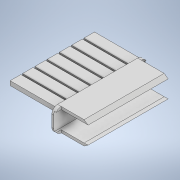
# Autodesk Inventor part: the whole thing
Saved by Autodesk Inventor 2020.2 (Build 242310000, 310)
## iProperties
Created: 2020-05-05
Part Number: the whole thing
Material: Generic
Document SubType Name: Modeling
Designer: Amaan Khalid
Density: 1 g/cm^3
Appearance: Default
Author: Amaan Khalid
Autodesk Inventor part; units mm, degrees
ref_plane "YZ Plane" through (0, 0, 0) normal (1, 0, 0) x (0, 1, 0)
ref_plane "XZ Plane" through (0, 0, 0) normal (0, 1, 0) x (-1, 0, 0)
ref_plane "XY Plane" through (0, 0, 0) normal (0, 0, 1) x (1, 0, 0)
sketch "Sketch1" plane through (0, 0, 0) normal (1, 0, 0) x (0, 1, 0)
  line L0 (-4.5658, 12.6718) -> (-17.2658, 12.6718)
  line L1 (-23.6158, 6.3218) -> (-23.6158, -82.5782)
  line L2 (-17.2658, -88.9282) -> (-4.5658, -88.9282)
  line L3 (1.7842, -82.5782) -> (1.7842, 6.3218)
  arc A0 (1.7842, 6.3218) -> (-4.5658, 12.6718) centre (-4.5658, 6.3218) ccw
  arc A1 (-17.2658, 12.6718) -> (-23.6158, 6.3218) centre (-17.2658, 6.3218) ccw
  arc A2 (-23.6158, -82.5782) -> (-17.2658, -88.9282) centre (-17.2658, -82.5782) ccw
  arc A3 (-4.5658, -88.9282) -> (1.7842, -82.5782) centre (-4.5658, -82.5782) ccw
  point P0 (0, 0)
  point P1 (1.7842, 12.6718)
  point P2 (-23.6158, -88.9282)
  point P3 (-23.6158, 12.6718)
  point P4 (1.7842, -88.9282)
  dimension "d0" = 25.4
  dimension "d1" = 101.6
  dimension "d4" = 6.35
  constraints: 8 end point, 8 point on circle, 8 point on line, 8 tangent, 4 centre point, 3 equal radius, 2 parallel, 1 horizontal, 1 perpendicular
  measures "d0" distance of point (1.784, -88.928) point (-23.616, -88.928)
  measures "d1" distance of point (-23.616, -88.928) point (-23.616, 12.672)
  measures "d4" radius of A0
extrude "Extrusion1" add sketch "Sketch1" along normal blind 4.064
sketch "Sketch2" plane through (4.064, 0, 0) normal (1, 0, 0) x (0, 0, -1)
  arc A0 (82.5782, -23.6158) -> (88.9282, -17.2658) centre (82.5782, -17.2658) ccw projected
  line L0 (-12.6718, -4.5658) -> (-12.6718, -17.2658) projected
  line L1 (82.5782, 1.7842) -> (-6.3218, 1.7842) projected
  line L2 (82.5782, -1.213) -> (-6.3218, -1.213)
  line L3 (-6.3218, -20.6186) -> (82.5782, -20.6186)
  line L4 (-6.3218, -20.6186) -> (82.5782, -20.6186)
  line L5 (82.5782, -20.6186) -> (82.5782, -23.6158)
  line L6 (82.5782, -23.6158) -> (-6.3218, -23.6158)
  line L7 (-6.3218, -23.6158) -> (-6.3218, -20.6186)
  line L8 (-6.3218, -1.213) -> (82.5782, -1.213)
  line L9 (82.5782, -1.213) -> (82.5782, 1.7842)
  line L10 (82.5782, 1.7842) -> (-6.3218, 1.7842)
  line L11 (-6.3218, 1.7842) -> (-6.3218, -1.213)
  point P0 (0, 0)
  dimension "d6" = 19.4056
  constraints: 20 end point, 5 parallel, 3 horizontal, 2 perpendicular
  measures "d6" distance of L3.start L2.end
extrude "Extrusion2" add sketch "Sketch2" along normal blind 25.4
sketch "Sketch3" plane through (4.064, -1.213, 6.3218) normal (0, 0, 1) x (1, 0, 0)
  line L0 (25.4, 2.9972) -> (25.4, 0) projected
  line L1 (25.4, 2.9972) -> (25.4, 0)
  line L2 (25.4, -19.4056) -> (25.4, -22.4028) projected
  line L3 (25.4, -22.4028) -> (29.8318, -19.2996)
  line L4 (25.4, -19.4056) -> (25.4, -22.4028)
  line L5 (0, 2.9972) -> (25.4, 2.9972) projected
  line L6 (25.4, 2.9972) -> (25.4, 0)
  line L7 (25.4, 2.9972) -> (29.8318, -0.106)
  line L8 (29.7989, -0.0829) -> (25.4, 0)
  line L9 (29.8318, -19.2996) -> (25.4, -19.4056)
  point P0 (-4.064, 1.213)
  dimension "d35" = 5.4102
  dimension "d36" = 55
  dimension "d37" = 5.4102
  dimension "d38" = 55
  constraints: 14 end point, 1 collinear, 1 perpendicular, 1 point on line, 1 vertical
  measures "d35" distance of L2.end L3.end
  measures "d36" angle of L7 L0
  measures "d37" distance of L0.start L7.end
  measures "d38" angle of L3 L2
sketch "Sketch4" plane through (0, 0, 0) normal (-1, 0, 0) x (0, 0, 1)
  arc A0 (12.6718, -4.5658) -> (6.3218, 1.7842) centre (6.3218, -4.5658) ccw projected
  line L0 (-5.4816, 0) -> (-17.3349, 0)
  line L1 (-17.3349, 0) -> (-17.3349, -4.7413)
  line L2 (-17.3349, -4.7413) -> (-5.4816, -4.7413)
  line L3 (-5.4816, -4.7413) -> (-5.4816, 0)
  line L4 (-30.9663, 0) -> (-19.1129, 0)
  line L5 (-19.1129, 0) -> (-19.1129, -4.7413)
  line L6 (-19.1129, -4.7413) -> (-30.9663, -4.7413)
  line L7 (-30.9663, -4.7413) -> (-30.9663, 0)
  line L8 (-32.7443, 0) -> (-44.5976, 0)
  line L9 (-44.5976, -4.7413) -> (-32.7443, -4.7413)
  line L10 (-32.7443, -4.7413) -> (-32.7443, 0)
  line L11 (-44.5976, 0) -> (-44.5976, -4.7413)
  arc A1 (-82.5782, 1.7842) -> (-88.9282, -4.5658) centre (-82.5782, -4.5658) ccw projected
  line L12 (-58.2289, -4.7413) -> (-58.2289, 0)
  line L13 (-58.2289, 0) -> (-46.3756, 0)
  line L14 (-46.3756, -4.7413) -> (-58.2289, -4.7413)
  line L15 (-46.3756, 0) -> (-46.3756, -4.7413)
  line L16 (-60.0069, 0) -> (-71.8603, 0)
  line L17 (-71.8603, 0) -> (-71.8603, -4.7413)
  line L18 (-71.8603, -4.7413) -> (-60.0069, -4.7413)
  line L19 (-60.0069, -4.7413) -> (-60.0069, 0)
  line L20 (-85.4916, 0) -> (-73.6383, 0)
  line L21 (-73.6383, 0) -> (-73.6383, -4.7413)
  line L22 (-85.4916, -4.7413) -> (-85.4916, 0)
  line L23 (-73.6383, -4.7413) -> (-85.4916, -4.7413)
  line L24 (-3.7036, 0) -> (8.1497, 0)
  line L25 (8.1497, 0) -> (8.1497, -4.7413)
  line L26 (8.1497, -4.7413) -> (-3.7036, -4.7413)
  line L27 (-3.7036, -4.7413) -> (-3.7036, 0)
  point P0 (0, 0)
  dimension "d47" = 1.778
  constraints: 56 end point, 2 parallel, 1 horizontal, 1 perpendicular
  measures "d47" distance between parallel lines of L5 L1
extrude "Extrusion4" add sketch "Sketch4" along normal blind 50.8
extrude "Extrusion6" add sketch "Sketch3" against normal up to surface (88.9 mm away)
sketch "Sketch8" plane through (0, -23.6158, -82.5782) normal (0, -1, 0) x (1, 0, 0)
  point P0 (0, 82.5782)
sketch "Sketch9" plane through (0, -23.6158, -82.5782) normal (0, -1, 0) x (1, 0, 0)
  line L0 (29.0881, 73.7677) -> (29.0881, 12.702) construction
  line L1 (29.0881, 12.702) -> (2.3767, 12.702) construction
  line L2 (2.3767, 12.702) -> (2.3767, 73.7677) construction
  line L3 (2.3767, 73.7677) -> (29.0881, 73.7677) construction
  point P0 (0, 82.5782)
  constraints: 2 other
emboss "Emboss2" [suppressed]
sketch "Sketch10" plane through (4.064, 0, 0) normal (1, 0, 0) x (0, 0, -1)
  line L0 (-6.3218, -20.6186) -> (82.5782, -20.6186) projected
  line L1 (82.5782, 1.7842) -> (82.5782, -1.213) projected
  line L2 (-6.3218, -1.213) -> (-6.3218, 1.7842) projected
  line L3 (82.5782, -1.213) -> (-6.3218, -1.213)
  line L4 (-6.3218, -20.6186) -> (82.5782, -20.6186)
  line L5 (82.5782, -20.6186) -> (87.9709, -20.6186)
  arc A0 (82.5782, -23.6158) -> (88.9282, -17.2658) centre (82.5782, -17.2658) ccw projected
  line L6 (82.5782, -1.213) -> (87.9709, -1.213)
  arc A1 (88.9282, -4.5658) -> (82.5782, 1.7842) centre (82.5782, -4.5658) ccw projected
  line L7 (-6.3218, -20.6186) -> (82.5782, -20.6186) projected
  line L8 (-6.3218, -20.6186) -> (-11.7145, -20.6186)
  arc A2 (-12.6718, -17.2658) -> (-6.3218, -23.6158) centre (-6.3218, -17.2658) ccw projected
  line L9 (-6.3218, -1.213) -> (-11.7145, -1.213)
  line L10 (87.9709, -1.213) -> (88.9282, -1.213)
  line L11 (88.9282, -1.213) -> (88.9282, -20.6186)
  line L12 (88.9282, -20.6186) -> (87.9709, -20.6186)
  line L13 (-11.7145, -20.6186) -> (-12.6718, -20.6186)
  line L14 (-12.6718, -20.6186) -> (-12.6718, -1.213)
  line L15 (-12.6718, -1.213) -> (-11.7145, -1.213)
  arc A3 (-6.3218, 1.7842) -> (-12.6718, -4.5658) centre (-6.3218, -4.5658) ccw projected
  point P0 (0, 0)
  point P1 (42.8061, -20.6186)
  point P2 (29.4692, -20.6186)
  point P3 (42.8061, -20.6186)
  constraints: 24 end point, 5 horizontal, 4 point on circle, 2 perpendicular, 1 point on line
extrude "Extrusion7" cut sketch "Sketch10" against normal blind 2.032 contours L8 A2 L14 A3 L9 L3 L6 A1 L11 A0 L5 L0 | L13 L14 A2 | A0 L11 L12 | L14 L15 A3 | A1 L10 L11
body "Solid1"
